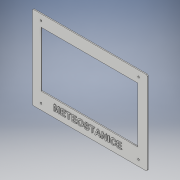
# Autodesk Inventor part: LCDv5-frontCover
Saved by Autodesk Inventor 2018 (Build 220112000, 112)
## iProperties
Created: 2017-11-06
Part Number: LCDv5-frontCover
Material: Generic
Document SubType Name: Modeling
Designer: WutchZone
Density: 1 g/cm^3
Appearance: Default
Author: WutchZone
Autodesk Inventor part; units mm, degrees
ref_plane "YZ Plane" through (0, 0, 0) normal (1, 0, 0) x (0, 1, 0)
ref_plane "XZ Plane" through (0, 0, 0) normal (0, 1, 0) x (-1, 0, 0)
ref_plane "XY Plane" through (0, 0, 0) normal (0, 0, 1) x (1, 0, 0)
sketch "Sketch1" plane through (0, 0, 0) normal (0, 0, 1) x (1, 0, 0)
  line L0 (92.45, -67.135) -> (-92.45, -67.135)
  line L1 (-92.45, -67.135) -> (-92.45, 67.135)
  line L2 (-92.45, 67.135) -> (92.45, 67.135)
  line L3 (92.45, 67.135) -> (92.45, -67.135)
  line L4 (92.45, -67.135) -> (-92.45, 67.135) construction
  line L5 (-92.45, -67.135) -> (92.45, 67.135) construction
  line L6 (77.45, -40.52) -> (-78.55, -40.52)
  line L7 (-78.55, -40.52) -> (-78.55, 48.48)
  line L8 (-78.55, 48.48) -> (77.45, 48.48)
  line L9 (77.45, 48.48) -> (77.45, -40.52)
  circle A0 centre (-78.45, 57.48) radius 1.5
  circle A1 centre (-78.45, -57.48) radius 1.5
  line L10 (0, 87.0056) -> (0, -123.2523) construction
  circle A2 centre (78.45, 57.48) radius 1.5
  circle A3 centre (78.45, -57.48) radius 1.5
  line L11 (-78.45, 57.48) -> (78.45, 57.48) construction
  line L12 (-78.45, 57.48) -> (-78.45, 67.135) construction
  line L13 (-78.45, -57.48) -> (-78.45, -67.135) construction
  point P0 (0, 0)
  point P1 (0, 67.135)
  point P2 (-78.55, 3.98)
  point P3 (-92.45, 0)
  point P4 (0, 57.48)
  dimension "d0" = 184.9
  dimension "d1" = 134.27
  dimension "d2" = 156
  dimension "d3" = 89
  dimension "d4" = 114.96
  dimension "d5" = 3
  dimension "d6" = 156.9
  dimension "d7" = 9
  dimension "d17" = 15
  dimension "d18" = 13.9
  constraints: 28 end point, 6 midpoint, 4 centre point, 4 parallel, 4 perpendicular, 3 horizontal, 3 vertical alignment, 2 point on line, 2 symmetric about line, 1 collinear, 1 equal radius, 1 vertical, 2 other
  measures "d0" distance of L1.end L2.end
  measures "d1" distance of L2.end L0.start
  measures "d2" distance of L7.end L8.end
  measures "d3" distance of L8.end L6.start
  measures "d4" distance of L13.start L11.start
  measures "d5" diameter of A0
  measures "d6" distance of L11.end L11.start
  measures "d7" distance from line of L11.start L8
  measures "d17" distance between parallel lines of L9 L3
  measures "d18" distance between parallel lines of L1 L7
extrude "Extrusion1" add sketch "Sketch1" along normal blind 1.6
fillet "Fillet1" radius 2 4 edges at (92.45, 67.135, 0.8) (-92.45, 67.135, 0.8) (92.45, -67.135, 0.8) (-92.45, -67.135, 0.8)
sketch "Sketch2" plane through (0, 0, 1.6) normal (0, 0, 1) x (1, 0, 0)
  line L0 (-58.4295, -47.2871) -> (67.3977, -47.2871) construction
  line L1 (67.3977, -47.2871) -> (67.3977, -69.3001) construction
  line L2 (67.3977, -69.3001) -> (-58.4295, -69.3001) construction
  line L3 (-58.4295, -69.3001) -> (-58.4295, -47.2871) construction
  line L4 (-54.0385, -55.8053) -> (-55.6133, -49.5447)
  line L5 (-55.6133, -49.5447) -> (-55.6133, -56.3329)
  spline S0 degree 2 poles (-55.6133, -56.3329) (-55.6133, -56.8915) (-56.1176, -57.4578) (-56.5288, -57.4578) knots 0 0 0 1 2 2 2
  spline S1 degree 2 poles (-56.5288, -57.4578) (-56.9322, -57.4578) (-57.4442, -56.8992) (-57.4442, -56.3329) knots 0 0 0 1 2 2 2
  line L6 (-57.4442, -56.3329) -> (-57.4442, -48.5517)
  spline S2 degree 2 poles (-57.4442, -48.5517) (-57.4442, -47.9077) (-56.777, -47.4578) (-56.2029, -47.4578) knots 0 0 0 1 2 2 2
  line L7 (-56.2029, -47.4578) -> (-55.5901, -47.4578)
  spline S3 degree 2 poles (-55.5901, -47.4578) (-55.0315, -47.4578) (-54.5272, -47.6595) (-54.2867, -48.1793) (-54.1316, -48.7689) knots 0 0 0 1 2 3 3 3
  line L8 (-54.1316, -48.7689) -> (-52.7041, -54.1529)
  line L9 (-52.7041, -54.1529) -> (-51.2766, -48.7689)
  spline S4 degree 2 poles (-51.2766, -48.7689) (-51.1215, -48.1793) (-50.881, -47.6595) (-50.3767, -47.4578) (-49.8181, -47.4578) knots 0 0 0 1 2 3 3 3
  line L10 (-49.8181, -47.4578) -> (-49.2053, -47.4578)
  spline S5 degree 2 poles (-49.2053, -47.4578) (-48.6312, -47.4578) (-47.964, -47.9077) (-47.964, -48.5517) knots 0 0 0 1 2 2 2
  line L11 (-47.964, -48.5517) -> (-47.964, -56.3329)
  spline S6 degree 2 poles (-47.964, -56.3329) (-47.964, -56.8915) (-48.4683, -57.4578) (-48.8872, -57.4578) knots 0 0 0 1 2 2 2
  spline S7 degree 2 poles (-48.8872, -57.4578) (-49.2829, -57.4578) (-49.7949, -56.8915) (-49.7949, -56.3329) knots 0 0 0 1 2 2 2
  line L12 (-49.7949, -56.3329) -> (-49.7949, -49.5447)
  line L13 (-49.7949, -49.5447) -> (-51.3697, -55.8053)
  spline S8 degree 2 poles (-51.3697, -55.8053) (-51.5249, -56.4182) (-51.7188, -56.9845) (-52.2386, -57.4578) (-52.7041, -57.4578) knots 0 0 0 1 2 3 3 3
  spline S9 degree 2 poles (-52.7041, -57.4578) (-53.0532, -57.4578) (-53.5342, -57.1552) (-53.8057, -56.6897) (-53.9609, -56.1157) (-54.0385, -55.8053) knots 0 0 0 1 2 3 4 4 4
  line L14 (-39.4458, -48.9939) -> (-43.9299, -48.9939)
  line L15 (-43.9299, -48.9939) -> (-43.9299, -51.4066)
  line L16 (-43.9299, -51.4066) -> (-39.8026, -51.4066)
  spline S10 degree 2 poles (-39.8026, -51.4066) (-39.3449, -51.4066) (-38.895, -51.8178) (-38.895, -52.1513) knots 0 0 0 1 2 2 2
  spline S11 degree 2 poles (-38.895, -52.1513) (-38.895, -52.4849) (-39.3372, -52.9116) (-39.8026, -52.9116) knots 0 0 0 1 2 2 2
  line L17 (-39.8026, -52.9116) -> (-43.9299, -52.9116)
  line L18 (-43.9299, -52.9116) -> (-43.9299, -55.7045)
  line L19 (-43.9299, -55.7045) -> (-39.2906, -55.7045)
  spline S12 degree 2 poles (-39.2906, -55.7045) (-38.8174, -55.7045) (-38.3441, -56.1389) (-38.3441, -56.5036) knots 0 0 0 1 2 2 2
  spline S13 degree 2 poles (-38.3441, -56.5036) (-38.3441, -56.8527) (-38.8174, -57.2871) (-39.2906, -57.2871) knots 0 0 0 1 2 2 2
  line L20 (-39.2906, -57.2871) -> (-44.6979, -57.2871)
  spline S14 degree 2 poles (-44.6979, -57.2871) (-45.3496, -57.2871) (-45.9159, -56.713) (-45.9159, -56.0691) knots 0 0 0 1 2 2 2
  line L21 (-45.9159, -56.0691) -> (-45.9159, -48.6758)
  spline S15 degree 2 poles (-45.9159, -48.6758) (-45.9159, -48.2491) (-45.6599, -47.706) (-45.1168, -47.4578) (-44.6979, -47.4578) knots 0 0 0 1 2 3 3 3
  line L22 (-44.6979, -47.4578) -> (-39.4458, -47.4578)
  spline S16 degree 2 poles (-39.4458, -47.4578) (-38.9648, -47.4578) (-38.5071, -47.8767) (-38.5071, -48.2258) knots 0 0 0 1 2 2 2
  spline S17 degree 2 poles (-38.5071, -48.2258) (-38.5071, -48.5749) (-38.9648, -48.9939) (-39.4458, -48.9939) knots 0 0 0 1 2 2 2
  line L23 (-30.3845, -49.1025) -> (-32.5567, -49.1025)
  line L24 (-32.5567, -49.1025) -> (-32.5567, -56.2475)
  spline S18 degree 2 poles (-32.5567, -56.2475) (-32.5567, -56.8604) (-33.1075, -57.4578) (-33.542, -57.4578) knots 0 0 0 1 2 2 2
  spline S19 degree 2 poles (-33.542, -57.4578) (-33.9842, -57.4578) (-34.5427, -56.8527) (-34.5427, -56.2475) knots 0 0 0 1 2 2 2
  line L25 (-34.5427, -56.2475) -> (-34.5427, -49.1025)
  line L26 (-34.5427, -49.1025) -> (-36.715, -49.1025)
  spline S20 degree 2 poles (-36.715, -49.1025) (-37.227, -49.1025) (-37.7235, -48.6525) (-37.7235, -48.2801) knots 0 0 0 1 2 2 2
  spline S21 degree 2 poles (-37.7235, -48.2801) (-37.7235, -47.9) (-37.2037, -47.4578) (-36.715, -47.4578) knots 0 0 0 1 2 2 2
  line L27 (-36.715, -47.4578) -> (-30.3845, -47.4578)
  spline S22 degree 2 poles (-30.3845, -47.4578) (-29.8647, -47.4578) (-29.3682, -47.9155) (-29.3682, -48.2801) knots 0 0 0 1 2 2 2
  spline S23 degree 2 poles (-29.3682, -48.2801) (-29.3682, -48.6525) (-29.8725, -49.1025) (-30.3845, -49.1025) knots 0 0 0 1 2 2 2
  line L28 (-21.7111, -48.9939) -> (-26.1952, -48.9939)
  line L29 (-26.1952, -48.9939) -> (-26.1952, -51.4066)
  line L30 (-26.1952, -51.4066) -> (-22.068, -51.4066)
  spline S24 degree 2 poles (-22.068, -51.4066) (-21.6102, -51.4066) (-21.1603, -51.8178) (-21.1603, -52.1513) knots 0 0 0 1 2 2 2
  spline S25 degree 2 poles (-21.1603, -52.1513) (-21.1603, -52.4849) (-21.6025, -52.9116) (-22.068, -52.9116) knots 0 0 0 1 2 2 2
  line L31 (-22.068, -52.9116) -> (-26.1952, -52.9116)
  line L32 (-26.1952, -52.9116) -> (-26.1952, -55.7045)
  line L33 (-26.1952, -55.7045) -> (-21.5559, -55.7045)
  spline S26 degree 2 poles (-21.5559, -55.7045) (-21.0827, -55.7045) (-20.6095, -56.1389) (-20.6095, -56.5036) knots 0 0 0 1 2 2 2
  spline S27 degree 2 poles (-20.6095, -56.5036) (-20.6095, -56.8527) (-21.0827, -57.2871) (-21.5559, -57.2871) knots 0 0 0 1 2 2 2
  line L34 (-21.5559, -57.2871) -> (-26.9632, -57.2871)
  spline S28 degree 2 poles (-26.9632, -57.2871) (-27.6149, -57.2871) (-28.1812, -56.713) (-28.1812, -56.0691) knots 0 0 0 1 2 2 2
  line L35 (-28.1812, -56.0691) -> (-28.1812, -48.6758)
  spline S29 degree 2 poles (-28.1812, -48.6758) (-28.1812, -48.2491) (-27.9252, -47.706) (-27.3822, -47.4578) (-26.9632, -47.4578) knots 0 0 0 1 2 3 3 3
  line L36 (-26.9632, -47.4578) -> (-21.7111, -47.4578)
  spline S30 degree 2 poles (-21.7111, -47.4578) (-21.2301, -47.4578) (-20.7724, -47.8767) (-20.7724, -48.2258) knots 0 0 0 1 2 2 2
  spline S31 degree 2 poles (-20.7724, -48.2258) (-20.7724, -48.5749) (-21.2301, -48.9939) (-21.7111, -48.9939) knots 0 0 0 1 2 2 2
  spline S32 degree 2 poles (-14.7057, -47.2871) (-13.1773, -47.2871) (-10.9818, -48.5284) (-9.8569, -50.817) (-9.8569, -52.3608) knots 0 0 0 1 2 3 3 3
  spline S33 degree 2 poles (-9.8569, -52.3608) (-9.8569, -53.5012) (-10.4698, -55.3631) (-11.7111, -56.7363) (-13.5032, -57.4578) (-14.6669, -57.4578) knots 0 0 0 1 2 3 4 4 4
  spline S34 degree 2 poles (-14.6669, -57.4578) (-15.815, -57.4578) (-17.6382, -56.713) (-18.8639, -55.3554) (-19.4846, -53.4547) (-19.4846, -52.3453) knots 0 0 0 1 2 3 4 4 4
  spline S35 degree 2 poles (-19.4846, -52.3453) (-19.4846, -51.2126) (-18.8329, -49.3197) (-17.5994, -47.9931) (-15.8306, -47.2871) (-14.7057, -47.2871) knots 0 0 0 1 2 3 4 4 4
  spline S36 degree 2 poles (-11.874, -52.3453) (-11.874, -51.2669) (-12.5722, -49.6843) (-13.8678, -48.8697) (-14.7057, -48.8697) knots 0 0 0 1 2 3 3 3
  spline S37 degree 2 poles (-14.7057, -48.8697) (-15.303, -48.8697) (-16.3116, -49.3197) (-17.0486, -50.1808) (-17.4675, -51.5152) (-17.4675, -52.3453) knots 0 0 0 1 2 3 4 4 4
  spline S38 degree 2 poles (-17.4675, -52.3453) (-17.4675, -53.1832) (-17.0486, -54.5408) (-16.2728, -55.433) (-15.272, -55.8752) (-14.6746, -55.8752) knots 0 0 0 1 2 3 4 4 4
  spline S39 degree 2 poles (-14.6746, -55.8752) (-13.9143, -55.8752) (-12.6343, -55.1071) (-11.874, -53.5167) (-11.874, -52.3453) knots 0 0 0 1 2 3 3 3
  spline S40 degree 2 poles (-0.687, -54.3391) (-0.687, -55.2313) (-1.6025, -56.651) (-3.3713, -57.4578) (-4.5893, -57.4578) knots 0 0 0 1 2 3 3 3
  spline S41 degree 2 poles (-4.5893, -57.4578) (-6.04, -57.4578) (-6.9865, -56.907) knots 0 0 0 1 1 1
  spline S42 degree 2 poles (-6.9865, -56.907) (-7.6537, -56.5113) (-8.4915, -55.1925) (-8.4915, -54.5641) knots 0 0 0 1 2 2 2
  spline S43 degree 2 poles (-8.4915, -54.5641) (-8.4915, -54.2072) (-7.995, -53.6874) (-7.6071, -53.6874) knots 0 0 0 1 2 2 2
  spline S44 degree 2 poles (-7.6071, -53.6874) (-7.2891, -53.6874) (-6.8546, -54.0908) (-6.6995, -54.4865) knots 0 0 0 1 2 2 2
  spline S45 degree 2 poles (-6.6995, -54.4865) (-6.5133, -54.9597) (-6.0788, -55.5881) (-5.2875, -55.9993) (-4.6436, -55.9993) knots 0 0 0 1 2 3 3 3
  spline S46 degree 2 poles (-4.6436, -55.9993) (-3.7592, -55.9993) (-2.6498, -55.1769) (-2.6498, -54.5563) knots 0 0 0 1 2 2 2
  spline S47 degree 2 poles (-2.6498, -54.5563) (-2.6498, -54.0676) (-3.2472, -53.4547) (-4.1936, -53.1288) (-4.9849, -52.9504) knots 0 0 0 1 2 3 3 3
  spline S48 degree 2 poles (-4.9849, -52.9504) (-6.04, -52.7022) (-7.4675, -52.035) (-8.3053, -50.8868) (-8.3053, -50.0412) knots 0 0 0 1 2 3 3 3
  spline S49 degree 2 poles (-8.3053, -50.0412) (-8.3053, -49.2266) (-7.4209, -47.9621) (-5.7452, -47.2871) (-4.6126, -47.2871) knots 0 0 0 1 2 3 3 3
  spline S50 degree 2 poles (-4.6126, -47.2871) (-3.7126, -47.2871) (-2.386, -47.7371) (-1.5171, -48.4818) (-1.1137, -49.2964) (-1.1137, -49.6843) knots 0 0 0 1 2 3 4 4 4
  spline S51 degree 2 poles (-1.1137, -49.6843) (-1.1137, -50.0412) (-1.618, -50.6153) (-1.9904, -50.6153) knots 0 0 0 1 2 2 2
  spline S52 degree 2 poles (-1.9904, -50.6153) (-2.3317, -50.6153) (-2.6886, -50.2739) (-2.8981, -49.886) knots 0 0 0 1 2 2 2
  spline S53 degree 2 poles (-2.8981, -49.886) (-3.1696, -49.3274) (-3.9143, -48.6991) (-4.7522, -48.6991) knots 0 0 0 1 2 2 2
  spline S54 degree 2 poles (-4.7522, -48.6991) (-5.5202, -48.6991) (-6.4667, -49.374) (-6.4667, -49.855) knots 0 0 0 1 2 2 2
  spline S55 degree 2 poles (-6.4667, -49.855) (-6.4667, -50.1498) (-6.1409, -50.5765) (-5.5823, -50.8868) (-5.0005, -51.0652) (-4.341, -51.2281) knots 0 0 0 1 2 3 4 4 4
  spline S56 degree 2 poles (-4.341, -51.2281) (-3.5109, -51.4221) (-2.1611, -51.8953) (-1.2146, -52.5703) (-0.687, -53.5943) (-0.687, -54.3391) knots 0 0 0 1 2 3 4 4 4
  line L37 (7.3812, -49.1025) -> (5.209, -49.1025)
  line L38 (5.209, -49.1025) -> (5.209, -56.2475)
  spline S57 degree 2 poles (5.209, -56.2475) (5.209, -56.8604) (4.6582, -57.4578) (4.2237, -57.4578) knots 0 0 0 1 2 2 2
  spline S58 degree 2 poles (4.2237, -57.4578) (3.7815, -57.4578) (3.223, -56.8527) (3.223, -56.2475) knots 0 0 0 1 2 2 2
  line L39 (3.223, -56.2475) -> (3.223, -49.1025)
  line L40 (3.223, -49.1025) -> (1.0507, -49.1025)
  spline S59 degree 2 poles (1.0507, -49.1025) (0.5387, -49.1025) (0.0422, -48.6525) (0.0422, -48.2801) knots 0 0 0 1 2 2 2
  spline S60 degree 2 poles (0.0422, -48.2801) (0.0422, -47.9) (0.562, -47.4578) (1.0507, -47.4578) knots 0 0 0 1 2 2 2
  line L41 (1.0507, -47.4578) -> (7.3812, -47.4578)
  spline S61 degree 2 poles (7.3812, -47.4578) (7.901, -47.4578) (8.3975, -47.9155) (8.3975, -48.2801) knots 0 0 0 1 2 2 2
  spline S62 degree 2 poles (8.3975, -48.2801) (8.3975, -48.6525) (7.8933, -49.1025) (7.3812, -49.1025) knots 0 0 0 1 2 2 2
  line L42 (15.8684, -56.17) -> (15.403, -54.9364)
  line L43 (15.403, -54.9364) -> (11.4076, -54.9364)
  line L44 (11.4076, -54.9364) -> (10.9344, -56.201)
  spline S63 degree 2 poles (10.9344, -56.201) (10.6628, -56.938) (10.2749, -57.4578) (9.8327, -57.4578) knots 0 0 0 1 2 2 2
  spline S64 degree 2 poles (9.8327, -57.4578) (9.4526, -57.4578) (8.8785, -56.907) (8.8785, -56.5579) knots 0 0 0 1 2 2 2
  spline S65 degree 2 poles (8.8785, -56.5579) (8.8785, -56.3562) (9.0104, -55.9295) (9.1656, -55.5493) knots 0 0 0 1 2 2 2
  line L45 (9.1656, -55.5493) -> (11.6791, -49.1568)
  spline S66 degree 2 poles (11.6791, -49.1568) (11.7877, -48.8852) (12.0903, -48.1095) (12.4317, -47.6052) (12.9902, -47.2871) (13.3936, -47.2871) knots 0 0 0 1 2 3 4 4 4
  spline S67 degree 2 poles (13.3936, -47.2871) (13.8126, -47.2871) (14.3711, -47.6052) (14.7125, -48.1017) (14.9452, -48.668) (15.1237, -49.149) knots 0 0 0 1 2 3 4 4 4
  line L46 (15.1237, -49.149) -> (17.6915, -55.495)
  spline S68 degree 2 poles (17.6915, -55.495) (17.9941, -56.2165) (17.9941, -56.5423) knots 0 0 0 1 1 1
  spline S69 degree 2 poles (17.9941, -56.5423) (17.9941, -56.8837) (17.4278, -57.4578) (17.0244, -57.4578) knots 0 0 0 1 2 2 2
  spline S70 degree 2 poles (17.0244, -57.4578) (16.7839, -57.4578) (16.4503, -57.2871) (16.2253, -57.0001) (15.9615, -56.4027) (15.8684, -56.17) knots 0 0 0 1 2 3 4 4 4
  line L47 (11.9274, -53.4469) -> (14.8677, -53.4469)
  line L48 (14.8677, -53.4469) -> (13.3859, -49.3895)
  line L49 (13.3859, -49.3895) -> (11.9274, -53.4469)
  line L50 (22.0515, -48.4818) -> (25.8762, -54.277)
  line L51 (25.8762, -54.277) -> (25.8762, -48.4275)
  spline S71 degree 2 poles (25.8762, -48.4275) (25.8762, -47.8534) (26.3649, -47.2871) (26.7839, -47.2871) knots 0 0 0 1 2 2 2
  spline S72 degree 2 poles (26.7839, -47.2871) (27.2106, -47.2871) (27.7071, -47.8534) (27.7071, -48.4275) knots 0 0 0 1 2 2 2
  line L52 (27.7071, -48.4275) -> (27.7071, -56.1622)
  spline S73 degree 2 poles (27.7071, -56.1622) (27.7071, -57.4578) (26.6365, -57.4578) knots 0 0 0 1 1 1
  spline S74 degree 2 poles (26.6365, -57.4578) (26.3649, -57.4578) (25.9383, -57.3026) (25.5581, -56.969) (25.24, -56.5191) (25.0771, -56.2863) knots 0 0 0 1 2 3 4 4 4
  line L53 (25.0771, -56.2863) -> (21.3455, -50.5532)
  line L54 (21.3455, -50.5532) -> (21.3455, -56.3174)
  spline S75 degree 2 poles (21.3455, -56.3174) (21.3455, -56.8837) (20.818, -57.4578) (20.4146, -57.4578) knots 0 0 0 1 2 2 2
  spline S76 degree 2 poles (20.4146, -57.4578) (19.9879, -57.4578) (19.4759, -56.8759) (19.4759, -56.3174) knots 0 0 0 1 2 2 2
  line L55 (19.4759, -56.3174) -> (19.4759, -48.7301)
  spline S77 degree 2 poles (19.4759, -48.7301) (19.4759, -48.2491) (19.5845, -47.9698) knots 0 0 0 1 1 1
  spline S78 degree 2 poles (19.5845, -47.9698) (19.7086, -47.6672) (20.306, -47.2871) (20.6473, -47.2871) knots 0 0 0 1 2 2 2
  spline S79 degree 2 poles (20.6473, -47.2871) (20.9111, -47.2871) (21.299, -47.4578) (21.586, -47.7603) (21.8886, -48.2258) (22.0515, -48.4818) knots 0 0 0 1 2 3 4 4 4
  line L56 (29.9724, -56.2398) -> (29.9724, -48.4973)
  spline S80 degree 2 poles (29.9724, -48.4973) (29.9724, -47.8922) (30.5232, -47.2871) (30.9576, -47.2871) knots 0 0 0 1 2 2 2
  spline S81 degree 2 poles (30.9576, -47.2871) (31.3998, -47.2871) (31.9584, -47.8845) (31.9584, -48.4973) knots 0 0 0 1 2 2 2
  line L57 (31.9584, -48.4973) -> (31.9584, -56.2398)
  spline S82 degree 2 poles (31.9584, -56.2398) (31.9584, -56.8527) (31.3998, -57.4578) (30.9576, -57.4578) knots 0 0 0 1 2 2 2
  spline S83 degree 2 poles (30.9576, -57.4578) (30.531, -57.4578) (29.9724, -56.8449) (29.9724, -56.2398) knots 0 0 0 1 2 2 2
  spline S84 degree 2 poles (42.5558, -54.1839) (42.5558, -54.6572) (42.0981, -55.7433) (41.105, -56.7984) (39.5612, -57.4578) (38.5372, -57.4578) knots 0 0 0 1 2 3 4 4 4
  spline S85 degree 2 poles (38.5372, -57.4578) (37.7614, -57.4578) (36.4813, -57.163) (35.4417, -56.5423) (35.0073, -56.0303) knots 0 0 0 1 2 3 3 3
  spline S86 degree 2 poles (35.0073, -56.0303) (34.6194, -55.5648) (34.0686, -54.4167) (33.7971, -53.1211) (33.7971, -52.3841) knots 0 0 0 1 2 3 3 3
  spline S87 degree 2 poles (33.7971, -52.3841) (33.7971, -51.1971) (34.4875, -49.3197) (35.7753, -47.9853) (37.5054, -47.2871) (38.4829, -47.2871) knots 0 0 0 1 2 3 4 4 4
  spline S88 degree 2 poles (38.4829, -47.2871) (39.6776, -47.2871) (41.5395, -48.2413) (42.5325, -49.6455) (42.5325, -50.2662) knots 0 0 0 1 2 3 3 3
  spline S89 degree 2 poles (42.5325, -50.2662) (42.5325, -50.6075) (42.0515, -51.1273) (41.7102, -51.1273) knots 0 0 0 1 2 2 2
  spline S90 degree 2 poles (41.7102, -51.1273) (41.3223, -51.1273) (40.9421, -50.7704) (40.7094, -50.3282) knots 0 0 0 1 2 2 2
  spline S91 degree 2 poles (40.7094, -50.3282) (40.3215, -49.5912) (39.2664, -48.8697) (38.4984, -48.8697) knots 0 0 0 1 2 2 2
  spline S92 degree 2 poles (38.4984, -48.8697) (37.2726, -48.8697) (35.8141, -50.7316) (35.8141, -52.4539) knots 0 0 0 1 2 2 2
  spline S93 degree 2 poles (35.8141, -52.4539) (35.8141, -53.6021) (36.458, -55.1226) (37.6372, -55.8752) (38.4286, -55.8752) knots 0 0 0 1 2 3 3 3
  spline S94 degree 2 poles (38.4286, -55.8752) (39.2897, -55.8752) (40.4767, -55.0218) (40.7792, -54.1994) knots 0 0 0 1 2 2 2
  spline S95 degree 2 poles (40.7792, -54.1994) (40.9033, -53.8115) (41.2757, -53.315) (41.6947, -53.315) knots 0 0 0 1 2 2 2
  spline S96 degree 2 poles (41.6947, -53.315) (42.0515, -53.315) (42.5558, -53.8115) (42.5558, -54.1839) knots 0 0 0 1 2 2 2
  line L58 (50.8258, -48.9939) -> (46.3417, -48.9939)
  line L59 (46.3417, -48.9939) -> (46.3417, -51.4066)
  line L60 (46.3417, -51.4066) -> (50.4689, -51.4066)
  spline S97 degree 2 poles (50.4689, -51.4066) (50.9266, -51.4066) (51.3766, -51.8178) (51.3766, -52.1513) knots 0 0 0 1 2 2 2
  spline S98 degree 2 poles (51.3766, -52.1513) (51.3766, -52.4849) (50.9344, -52.9116) (50.4689, -52.9116) knots 0 0 0 1 2 2 2
  line L61 (50.4689, -52.9116) -> (46.3417, -52.9116)
  line L62 (46.3417, -52.9116) -> (46.3417, -55.7045)
  line L63 (46.3417, -55.7045) -> (50.9809, -55.7045)
  spline S99 degree 2 poles (50.9809, -55.7045) (51.4542, -55.7045) (51.9274, -56.1389) (51.9274, -56.5036) knots 0 0 0 1 2 2 2
  spline S100 degree 2 poles (51.9274, -56.5036) (51.9274, -56.8527) (51.4542, -57.2871) (50.9809, -57.2871) knots 0 0 0 1 2 2 2
  line L64 (50.9809, -57.2871) -> (45.5736, -57.2871)
  spline S101 degree 2 poles (45.5736, -57.2871) (44.922, -57.2871) (44.3556, -56.713) (44.3556, -56.0691) knots 0 0 0 1 2 2 2
  line L65 (44.3556, -56.0691) -> (44.3556, -48.6758)
  spline S102 degree 2 poles (44.3556, -48.6758) (44.3556, -48.2491) (44.6116, -47.706) (45.1547, -47.4578) (45.5736, -47.4578) knots 0 0 0 1 2 3 3 3
  line L66 (45.5736, -47.4578) -> (50.8258, -47.4578)
  spline S103 degree 2 poles (50.8258, -47.4578) (51.3068, -47.4578) (51.7645, -47.8767) (51.7645, -48.2258) knots 0 0 0 1 2 2 2
  spline S104 degree 2 poles (51.7645, -48.2258) (51.7645, -48.5749) (51.3068, -48.9939) (50.8258, -48.9939) knots 0 0 0 1 2 2 2
  point P0 (0, 0)
  constraints: 2 other
extrude "Extrusion2" add sketch "Sketch2" along normal blind 1
body "Solid1"
